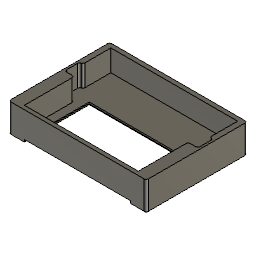
thermometer aa battery mod (Autodesk Fusion 360 design; units mm, degrees)
Autodesk Fusion 360 part; units mm, degrees
sketch "Sketch1" plane through (0, 0, 0) normal (0, 0, 1) x (1, 0, 0)
  line L0 (-22.5, -10) -> (22.5, -10)
  line L1 (22.5, -10) -> (22.5, 16)
  line L2 (22.5, 16) -> (-22.5, 16)
  line L3 (-22.5, 16) -> (-22.5, -10)
  line L4 (-29.5, 33) -> (29.5, 33)
  line L5 (29.5, 33) -> (29.5, 16)
  line L6 (29.5, 16) -> (-29.5, 16)
  line L7 (-29.5, 16) -> (-29.5, 33)
  line L8 (-32, 35) -> (32, 35)
  line L9 (32, 35) -> (32, -12)
  line L10 (32, -12) -> (-32, -12)
  line L11 (-32, -12) -> (-32, 35)
  line L12 (-22.5, 16) -> (-26.5, 16)
  line L13 (22.5, 16) -> (26.5, 16)
  line L14 (-26.5, 16) -> (-26.5, -10)
  line L15 (-26.5, -10) -> (-22.5, -10)
  line L16 (22.5, -10) -> (26.5, -10)
  line L17 (26.5, -10) -> (26.5, 16)
  dimension "d1" = 45
  dimension "d2" = 26
  dimension "d3" = 59
  dimension "d4" = 17
  dimension "d7" = 4
  dimension "d8" = 4
  dimension "d9" = 4
  constraint horizontal L0
  constraint vertical L1
  constraint horizontal L2
  constraint vertical L3
  constraint horizontal L4
  constraint vertical L5
  constraint horizontal L6
  constraint vertical L7
  constraint horizontal L8
  constraint vertical L9
  constraint horizontal L10
  constraint vertical L11
  constraint perpendicular L7 L12
  constraint perpendicular L1 L13
  constraint perpendicular L6 L14
  constraint perpendicular L3 L15
  constraint perpendicular L1 L16
  measures "d1" distance of L0.start L0.end
  measures "d2" distance of L0.start L2.end
  measures "d3" distance of L4.start L4.end
  measures "d4" distance of L4.start L6.end
  measures "d7" distance of L2.end L12.end
  measures "d8" distance of L1.end L13.end
  measures "d9" distance of L0.end L16.end
extrude "Extrude1" add sketch "Sketch1" along normal blind 1.5 from surface at 0.5 contours L3 L6 L12 L14 L15 | L1 L6 L13 L16 L17 | L2 L4 L5 L6 L7 L12 L13 | L8 L9 L10 L11
extrude "Extrude2" add sketch "Sketch1" along normal blind 12
sketch "Sketch2" plane through (0, 0, 0.5) normal (0, 0, -1) x (1, 0, 0)
  line L0 (32, 12) -> (-32, 12)
  line L1 (-32, 12) -> (-32, -35)
  line L2 (-32, -35) -> (32, -35)
  line L3 (32, -35) -> (32, 12)
  line L4 (-22.5, 10) -> (-26.5, 10)
  line L5 (22.5, 10) -> (22.5, -16)
  line L6 (22.5, -16) -> (-22.5, -16)
  line L7 (-22.5, -16) -> (-22.5, 10)
  line L8 (-24.5, -18) -> (-24.5, 12)
  line L9 (-24.5, 12) -> (24.5, 12)
  line L10 (24.5, 12) -> (24.5, -18)
  line L11 (24.5, -18) -> (-24.5, -18)
  line L12 (-26.5, 10) -> (-26.5, -16)
  line L13 (-26.5, -16) -> (-29.5, -16)
  line L14 (-29.5, -16) -> (-29.5, -33)
  line L15 (-29.5, -33) -> (29.5, -33)
  line L16 (29.5, -33) -> (29.5, -16)
  line L17 (29.5, -16) -> (26.5, -16)
  line L18 (26.5, -16) -> (26.5, 10)
  line L19 (26.5, 10) -> (22.5, 10)
  line L20 (-26.5, -16) -> (-26.5, 10)
  line L21 (-26.5, 10) -> (26.5, 10)
  line L22 (26.5, 10) -> (26.5, -16)
  line L23 (26.5, -16) -> (29.5, -16)
  line L24 (29.5, -16) -> (29.5, -33)
  line L25 (29.5, -33) -> (-29.5, -33)
  line L26 (-29.5, -33) -> (-29.5, -16)
  line L27 (-29.5, -16) -> (-26.5, -16)
  constraint parallel L7 L8
  constraint parallel L4 L9
  constraint parallel L5 L10
  constraint parallel L6 L11
extrude "Extrude3" add sketch "Sketch2" along normal blind 2 contours L0 L1 L2 L3 L4 L8 L10 L12 L13 L14 L15 L16 L17 L18 L19 L20 L21 L22 L23 L24 L25 L26 L27 | L4 L8 L10 L11 L12 L13 L14 L15 L16 L17 L18 L19 L20 L21 L22 L23 L24 L25 L26 L27
fillet "Fillet1" radius 1 2 edges at (-26.5, 16, 7) (26.5, 16, 7)
fillet "Fillet2" radius 1 4 edges at (-32, 35, 5.25) (-32, -12, 5.25) (32, -12, 5.25) (32, 35, 5.25)
move_face "OffsetFaces1" offset -0.2 7 faces at (-22.5, 7.3333, 1) (7.5, 16, 1) (22.5, -1.3333, 1) (7.5, -10, 8.6667) (24.5, 8.6667, -0.3333) (8.1667, 18, -0.1667) (-24.5, 8.6667, -0.3333)
box "BoxPrimitive1" add length 2.05 width 50 height 0.2 placed x (0, -1, 0) y (-1, 0, 0) z (0, 0, -1) at (24.75, 18.25, 0.5)
sketch "Sketch4" plane through (0, 0, 12) normal (0, 0, 1) x (-1, 0, 0)
  arc A0 (-32, -34) -> (-31, -35) centre (-31, -34) ccw
  line L0 (-31, -35) -> (31, -35)
  arc A1 (31, -35) -> (32, -34) centre (31, -34) ccw
  line L1 (32, -34) -> (32, 11)
  arc A2 (32, 11) -> (31, 12) centre (31, 11) ccw
  line L2 (31, 12) -> (-31, 12)
  arc A3 (-31, 12) -> (-32, 11) centre (-31, 11) ccw
  line L3 (-32, 11) -> (-32, -34)
  arc A4 (-27.5, -16) -> (-26.5, -15) centre (-27.5, -15) ccw
  line L4 (-26.5, -15) -> (-26.5, 10.2)
  line L5 (-26.5, 10.2) -> (26.5, 10.2)
  line L6 (26.5, 10.2) -> (26.5, -15)
  arc A5 (26.5, -15) -> (27.5, -16) centre (27.5, -15) ccw
  line L7 (27.5, -16) -> (29.5, -16)
  line L8 (29.5, -16) -> (29.5, -33)
  line L9 (29.5, -33) -> (-29.5, -33)
  line L10 (-29.5, -33) -> (-29.5, -16)
  line L11 (-29.5, -16) -> (-27.5, -16)
  line L12 (31, -20) -> (-31, -20)
  line L13 (-31, -20) -> (-31, -13)
  line L14 (-31, -13) -> (31, -13)
  line L15 (31, -13) -> (31, -20)
  dimension "d25" = 62
  constraint horizontal L12
  constraint vertical L13
  constraint horizontal L14
  constraint vertical L15
  measures "d25" distance of L12.start L12.end
extrude "Extrude4" cut sketch "Sketch4" against normal blind 10 contours A4 L4 L10 L11 L12 L13 L14 | L6 A5 L7 L8 L12 L14 L15
fillet "Fillet3" radius 1 6 edges at (29.5, 20, 7) (-29.5, 20, 7) (-31, 20, 7) (-31, 13, 7) (31, 20, 7) (31, 13, 7)
fillet "Fillet4" radius 1 2 edges at (-26.5, 13, 7) (26.5, 13, 7)
chamfer "Chamfer1" distance 0.4 angle 45 12 edges at (24.7, 3.1, -1.5) (0, 18.2, -1.5) (-24.7, 3.1, -1.5) (-27.85, -12, -1.5) (-31.7071, -11.7071, -1.5) (-32, 11.5, -1.5) (-31.7071, 34.7071, -1.5) (0, 35, -1.5) (31.7071, 34.7071, -1.5) (32, 11.5, -1.5) (31.7071, -11.7071, -1.5) (27.85, -12, -1.5)
chamfer "Chamfer1" distance 1 angle 45 4 edges at (-22.7, 3, 0.5) (0, -10.2, 0) (0, 16.2, 0.3) (22.7, 3, 0.5)
